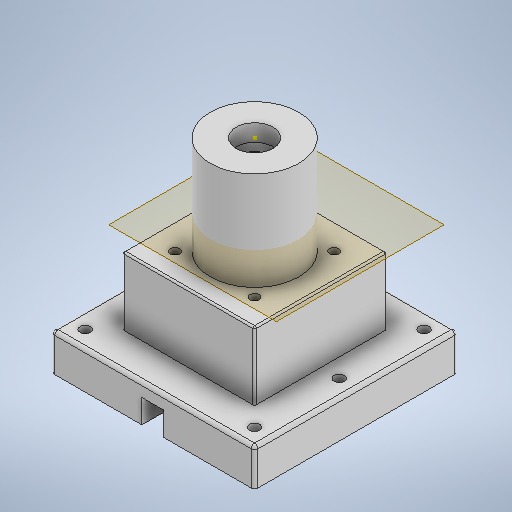
# Autodesk Inventor part: Eslabón1
Saved by Autodesk Inventor 2025.1 (Build 291241000, 241)
## iProperties
Created: 2024-12-06
Part Number: Eslabón1
Material: Generic
Document SubType Name: Modeling
Designer: Cristhian Vigo
Density: 1 g/cm^3
Appearance: Default
Author: Cristhian Vigo
Autodesk Inventor part; units mm, degrees
note: some values were not read from the file. Chosen so that the rebuilt part matches the saved one: second side of "Extrusion3"; second side of "Extrusion4".
ref_plane "YZ Plane" through (0, 0, 0) normal (1, 0, 0) x (0, 1, 0)
ref_plane "XY Plane" through (0, 0, 0) normal (0, 0, 1) x (1, 0, 0)
sketch "Sketch1" plane through (0, 0, 0) normal (0, 1, 0) x (-1, 0, 0)
  line L0 (-60, -60) -> (60, -60)
  line L1 (60, -60) -> (60, 60)
  line L2 (60, 60) -> (-60, 60)
  line L3 (-60, 60) -> (-60, -60)
  line L4 (-60, -60) -> (60, 60) construction
  line L5 (60, -60) -> (-60, 60) construction
  line L6 (-29, -29) -> (29, 29) construction
  line L7 (28, -28) -> (-28, 28) construction
  line L8 (-36.5, -36.5) -> (36.5, 36.5) construction
  line L9 (36.5, -36.5) -> (-36.5, 36.5) construction
  line L10 (-39, -39) -> (39, 39) construction
  line L11 (33.9, -33.9) -> (-33.9, 33.9) construction
  line L12 (-24.8, -24.8) -> (24.8, 24.8) construction
  line L13 (39.8, -39.8) -> (-39.8, 39.8) construction
  line L14 (-39, -39) -> (39, -39)
  line L15 (39, -39) -> (39, 39)
  line L16 (39, 39) -> (-39, 39)
  line L17 (-39, 39) -> (-39, -39)
  line L18 (-39, -39) -> (39, 39) construction
  line L19 (39, -39) -> (-39, 39) construction
  line L20 (-29, -29) -> (29, -29)
  line L21 (29, -29) -> (29, 29)
  line L22 (29, 29) -> (-29, 29)
  line L23 (-29, 29) -> (-29, -29)
  line L24 (-29, -29) -> (29, 29) construction
  line L25 (29, -29) -> (-29, 29) construction
  point P0 (0, 0)
  dimension "d0" = 120
  dimension "d1" = 120
  dimension "d13" = 78
  dimension "d14" = 78
  dimension "Largo_PaP" = 58
  dimension "Ancho_PaP" = 58
  constraints: 52 end point, 14 midpoint, 6 parallel, 3 horizontal, 3 perpendicular, 1 point on line
  measures "d0" distance of L2.end L1.end
  measures "d1" distance of L1.end L0.end
  measures "d13" distance of L16.end L10.end
  measures "d14" distance of L10.end L14.end
  measures "Largo_PaP" distance of L22.end L6.end
  measures "Ancho_PaP" distance of L6.end L20.end
extrude "Extrusion1" add sketch "Sketch1" along normal blind 22 contours L3 L2 L1 L0
extrude "Extrusion2" add sketch "Sketch1" along normal blind 62 contours L17 L16 L15 L14
sketch "Sketch2" plane through (0, 22, 0) normal (0, 1, 0) x (1, 0, 0)
  line L0 (-60, 60) -> (-60, -60) projected
  line L1 (60, -60) -> (60, 60) projected
  line L2 (-60, -60) -> (60, -60) projected
  line L3 (60, 60) -> (-60, 60) projected
  line L4 (50, 50) -> (-50, 50)
  line L5 (-50, 50) -> (-50, -50)
  line L6 (-50, -50) -> (50, -50)
  line L7 (50, -50) -> (50, 50)
  line L8 (50, 50) -> (-50, -50) construction
  line L9 (-50, 50) -> (50, -50) construction
  point P0 (50, 0)
  point P1 (0, 50)
  point P2 (-50, 0)
  dimension "d82" = 100
  dimension "d83" = 100
  constraints: 12 end point, 4 coincident, 3 midpoint, 2 horizontal, 2 parallel, 1 perpendicular, 1 vertical
  measures "d82" distance of L6.end L5.end
  measures "d83" distance of L5.end L4.end
hole "Hole1" at (-50, 22, 50) at (50, 22, 50) at (50, 22, -50) at (0, 22, -50) at (-50, 22, -50) at (-50, 22, 0) at (50, 22, 0) direction (0, -1, 0) diameter 6.1 end through all
sketch "Sketch3" plane through (0, 62, 0) normal (0, 1, 0) x (1, 0, 0)
  line L0 (29, -29) -> (-29, -29) projected
  line L1 (29, 29) -> (-29, 29)
  line L2 (-29, 29) -> (-29, -29)
  line L3 (-29, -29) -> (29, -29)
  line L4 (29, -29) -> (29, 29)
  line L5 (29, 29) -> (-29, -29) construction
  line L6 (-29, 29) -> (29, -29) construction
  line L7 (14, -14) -> (-14, 14) construction
  line L8 (-14, -14) -> (14, 14) construction
  line L9 (19, -19) -> (-19, 19) construction
  line L10 (-19, -19) -> (19, 19) construction
  circle A0 centre (0, 0) radius 19.15
  dimension "d56" = 38.3
  constraints: 20 end point, 4 midpoint, 2 parallel, 1 centre point, 1 coincident, 1 horizontal, 1 perpendicular
  measures "d56" diameter of A0
extrude "Extrusion3" add sketch "Sketch3" against normal blind 8
fillet "Fillet1" radius 2 8 edges at (0, 22, 60) (-60, 22, 0) (60, 22, 0) (0, 22, -60) (60, 11, 60) (-60, 11, 60) (60, 11, -60) (-60, 11, -60)
fillet "Fillet2" radius 1 8 edges at (0, 62, 39) (39, 62, 0) (0, 62, -39) (-39, 62, 0) (-39, 42, -39) (39, 42, -39) (-39, 42, 39) (39, 42, 39)
sketch "Sketch4" plane through (0, 62, 0) normal (0, 1, 0) x (1, 0, 0)
  line L0 (39, -38) -> (39, 38) projected
  line L1 (-38, -39) -> (38, -39) projected
  line L2 (0, -10.7148) -> (0, 11.656) construction
  line L3 (7.4793, 0) -> (-11.1938, 0) construction
  line L4 (28, 28) -> (-28, 28)
  line L5 (-28, 28) -> (-28, -28)
  line L6 (-28, -28) -> (28, -28)
  line L7 (28, -28) -> (28, 28)
  line L8 (28, 28) -> (-28, -28) construction
  line L9 (-28, 28) -> (28, -28) construction
  point P0 (0, 0)
  point P1 (23.5, -23.5)
  point P2 (-23.5, -23.5)
  point P3 (23.5, 23.5)
  point P4 (-23.5, 23.5)
  dimension "d53" = 56
  dimension "d54" = 56
  dimension "d57" = 47
  dimension "d58" = 47
  constraints: 16 end point, 3 symmetric about line, 2 horizontal, 2 midpoint, 2 parallel, 1 perpendicular, 1 point on line, 1 vertical
  measures "d53" distance of L6.end L5.end
  measures "d54" distance of L5.end L4.end
  measures "d57" distance of point (23.5, -23.5) point (-23.5, -23.5)
  measures "d58" distance of point (-23.5, 23.5) point (-23.5, -23.5)
hole "Hole2" at (-23.5, 62, 23.5) at (23.5, 62, 23.5) at (23.5, 62, -23.5) at (-23.5, 62, -23.5) direction (0, -1, 0) diameter 5.5 end through all
sketch "Sketch6" plane through (0, 62, 0) normal (0, 1, 0) x (1, 0, 0)
  circle A0 centre (0, 0) radius 19.15
  circle A1 centre (0, 0) radius 10
  dimension "d59" = 20
  dimension "d60" = 38.3
  constraints: 2 centre point, 2 coincident
  measures "d59" diameter of A1
  measures "d60" diameter of A0
extrude "Extrusion4" add sketch "Sketch6" against normal blind 5
sketch "Sketch12" plane through (0, 62, 0) normal (0, 1, 0) x (1, 0, 0)
  circle A0 centre (0, 0) radius 26.15
  circle A1 centre (0, 0) radius 10
  dimension "d85" = 52.3
  constraints: 2 centre point, 1 coincident, 1 other
  measures "d85" diameter of A0
extrude "Extrusion9" add sketch "Sketch12" along normal blind 28
sketch "Sketch13" plane through (0, 90, 0) normal (0, 1, 0) x (1, 0, 0)
  circle A0 centre (0, 0) radius 4.5
  circle A1 centre (0, 0) radius 10 projected
  circle A2 centre (0, 0) radius 26.15
  dimension "d88" = 9
  constraints: 2 centre point, 2 coincident, 1 other
  measures "d88" diameter of A0
extrude "Extrusion10" add sketch "Sketch13" along normal blind 20 contours A1 | A2
sketch "Sketch9" plane through (-58, 0, 60) normal (0, 0, 1) x (1, 0, 0)
  line L0 (0, 0) -> (0, 20) construction
  line L1 (0, 0) -> (116, 0) construction
  line L2 (0, 0) -> (116, 0) construction
  line L3 (64.5, -14) -> (51.5, -14)
  line L4 (51.5, -14) -> (51.5, 14)
  line L5 (51.5, 14) -> (64.5, 14)
  line L6 (64.5, 14) -> (64.5, -14)
  line L7 (64.5, -14) -> (51.5, 14) construction
  line L8 (51.5, -14) -> (64.5, 14) construction
  point P0 (58, 0)
  dimension "d77" = 13
  dimension "d78" = 28
  constraints: 14 end point, 2 horizontal, 2 midpoint, 2 parallel, 1 perpendicular
  measures "d77" distance of L4.end L5.end
  measures "d78" distance of L3.end L4.end
extrude "Extrusion8" cut sketch "Sketch9" against normal up to surface (31 mm away)
sketch "Sketch14" plane through (0, 110, 0) normal (0, 1, 0) x (1, 0, 0)
  circle A0 centre (0, 0) radius 10.9
  circle A1 centre (0, 0) radius 26.15
  dimension "d91" = 21.8
  constraints: 2 centre point, 2 coincident, 1 other
  measures "d91" diameter of A0
extrude "Extrusion11" add sketch "Sketch14" along normal blind 10
ref_plane "Work Plane3" through (0, 81.25, 0) normal (0, 1, 0) x (-1, 0, 0)
sketch "Sketch15" plane through (0, 120, 0) normal (0, 1, 0) x (1, 0, 0)
  point P0 (0, 0)
equation "\"Largo_PaP\" = Ancho_PaP"
body "Solid1"
